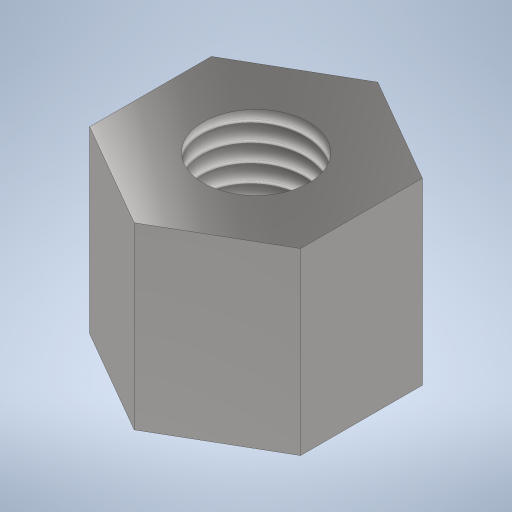
# Autodesk Inventor part: Spacer
Saved by Autodesk Inventor 2023.1 (Build 271208000, 208)
## iProperties
Created: 2023-11-19
Part Number: Spacer
Material: Steel, Mild
Document SubType Name: Modeling
Designer: JansenL
Density: 7.85 g/cm^3
Appearance: Semi-Polished
Author: JansenL
Autodesk Inventor part; units mm, degrees
ref_plane "YZ Plane" through (0, 0, 0) normal (1, 0, 0) x (0, 1, 0)
ref_plane "XZ Plane" through (0, 0, 0) normal (0, 1, 0) x (-1, 0, 0)
ref_plane "XY Plane" through (0, 0, 0) normal (0, 0, 1) x (1, 0, 0)
sketch "Sketch1" plane through (0, 0, 0) normal (0, 1, 0) x (-1, 0, 0)
  line L0 (0, 3.4641) -> (3, 1.7321)
  line L1 (3, 1.7321) -> (3, -1.7321)
  line L2 (3, -1.7321) -> (0, -3.4641)
  line L3 (0, -3.4641) -> (-3, -1.7321)
  line L4 (-3, -1.7321) -> (-3, 1.7321)
  line L5 (-3, 1.7321) -> (0, 3.4641)
  circle A0 centre (0, 0) radius 1.5
  line L6 (0, -4.8497) -> (0, 4.8497) projected
  dimension "d0" = 3
  dimension "d1" = 6
  constraints: 12 end point, 2 coincident, 1 centre point, 1 parallel, 13 other
  measures "d0" diameter of A0
  measures "d1" distance between parallel lines of L4 L1
extrude "Extrusion1" add sketch "Sketch1" along normal blind 5.1 contours L6 A0 L3 L4 L5 | L0 L1 L2 L6 A0
thread "Thread1" size "M3x0.5" class "6H" standard "ANSI Metric M Profile" full length
body "Solid1"
